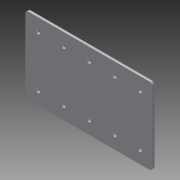
# Autodesk Inventor part: Support for Connect Arm to Funnel  (Custom)
Saved by Autodesk Inventor 2014 (Build 180170000, 170)
## iProperties
Created: 2014-01-07
Part Number: Support for Connect Arm to Funnel  (Custom)
Material: Aluminum 6061
Document SubType Name: Sheet Metal
Designer: Michael
Density: 2.71 g/cm^3
Sheet Metal Rule: Default
Appearance: Aluminum - Flat
Mass: 35.4111 g
Surface Area: 122.958 cm^2
Volume: 13.0668 cm^3
Author: Michael
Autodesk Inventor part; units mm, degrees
ref_plane "YZ Plane" through (0, 0, 0) normal (1, 0, 0) x (0, 1, 0)
ref_plane "XZ Plane" through (0, 0, 0) normal (0, 1, 0) x (-1, 0, 0)
ref_plane "XY Plane" through (0, 0, 0) normal (0, 0, 1) x (1, 0, 0)
sketch "Sketch1" plane through (0, 0, 0) normal (0, 0, 1) x (1, 0, 0)
  line L0 (0, 0) -> (127, 0)
  line L1 (127, 0) -> (127, 76.2)
  line L2 (127, 76.2) -> (0, 76.2)
  line L3 (0, 76.2) -> (0, 0)
  line L4 (0, 76.2) -> (127, 76.2) construction
  line L5 (127, 76.2) -> (127, 50.8) construction
  line L6 (127, 50.8) -> (0, 50.8) construction
  line L7 (0, 50.8) -> (0, 76.2) construction
  circle A0 centre (114.3, 63.5) radius 2.0828
  circle A1 centre (88.9, 63.5) radius 2.0828
  circle A2 centre (63.5, 63.5) radius 2.0828
  line L8 (0, 38.1) -> (127, 38.1) construction
  circle A3 centre (114.3, 12.7) radius 2.0828
  circle A4 centre (88.9, 12.7) radius 2.0828
  circle A5 centre (63.5, 12.7) radius 2.0828
  circle A6 centre (38.1, 63.5) radius 2.0828
  circle A7 centre (12.7, 63.5) radius 2.0828
  circle A8 centre (38.1, 12.7) radius 2.0828
  circle A9 centre (12.7, 12.7) radius 2.0828
  dimension "d0" = 127
  dimension "d1" = 76.2
  dimension "d2" = 25.4
  dimension "d3" = 4.1656
  dimension "d4" = 12.7
  dimension "d7" = 25.4
  dimension "d12" = 12.7
  measures "d0" distance of L2.end L1.end
  measures "d1" distance of L1.end L0.end
  measures "d2" distance of L4.end L5.end
  measures "d3" diameter of A0
  measures "d4" distance from line of L2 A0.centre
  measures "d7" distance of A0.centre A1.centre
  measures "d12" distance from line of L1 A0.centre
extrude "Plate1" add sketch "Sketch1" along normal blind 2.286
fillet "Fillet1" radius 3.175 4 edges at (127, 76.2, 1.143) (0, 76.2, 1.143) (127, 0, 1.143) (0, 0, 1.143)
equation "\"BendRadius\" = Thickness"
equation "\"BendReliefWidth\" = Thickness"
equation "\"BendReliefDepth\" = 0.5 * Thickness"
equation "\"CornerReliefSize\" = 4 * Thickness"
equation "\"MinimumRemnant\" = 2 * Thickness"
equation "\"TransitionRadius\" = BendRadius"
equation "\"JacobiRadiusSize\" = BendRadius"
equation "\"GapSize\" = Thickness"
equation "\"d13\" = BendRadius"
equation "\"Thickness\" = 2.286"
body "Solid1"
